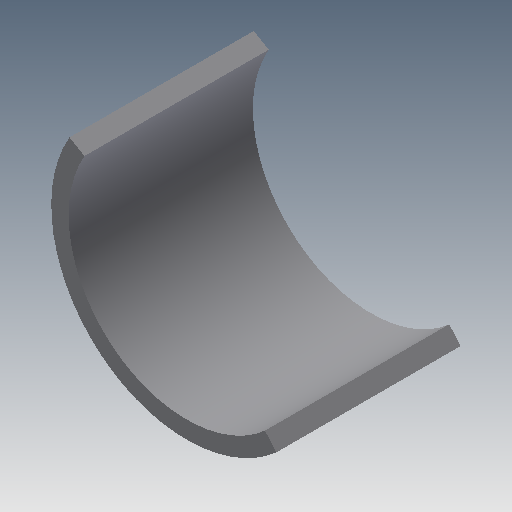
# Autodesk Inventor part: WeldExer_Guard_Plate
Saved by Autodesk Inventor 2020.1 (Build 241239000, 239)
## iProperties
Created: 2005-02-10
Part Number: WeldExer_Guard_Plate
Document SubType Name: Modeling
Designer: Dale Schneider
Manufacturer: Standard
Standards Organization: Custom
Stock Number: WeldExer_Guard_Plate
Density: 1 g/cm^3
Material: Generic
Appearance: Default
Author: Dale Schneider
Autodesk Inventor part; units mm, degrees
ref_plane "YZ Plane" through (0, 0, 0) normal (1, 0, 0) x (0, 1, 0)
ref_plane "XZ Plane" through (0, 0, 0) normal (0, 1, 0) x (-1, 0, 0)
ref_plane "XY Plane" through (0, 0, 0) normal (0, 0, 1) x (1, 0, 0)
sketch "Sketch1" plane through (0, 0, 0) normal (0, 0, 1) x (1, 0, 0)
  circle A0 centre (0, 0) radius 12.5
  circle A1 centre (0, 0) radius 10.8984
  line L0 (-9.4395, 5.4471) -> (-10.8267, 6.2476)
  line L1 (7.2139, -8.1691) -> (8.274, -9.3696)
  line L2 (0, 0) -> (-9.4395, 5.4471) construction
  line L3 (0, 0) -> (7.2139, -8.1691) construction
  dimension "d0" = 25
  constraints: 8 end point, 4 point on circle, 2 centre point, 2 coincident, 2 collinear
  measures "d0" diameter of A0
extrude "Extrusion1" add sketch "Sketch1" along normal blind 17 contours L0 A1 L1 A0 picked at (-10.7498, 5.084)
body "Solid1"
